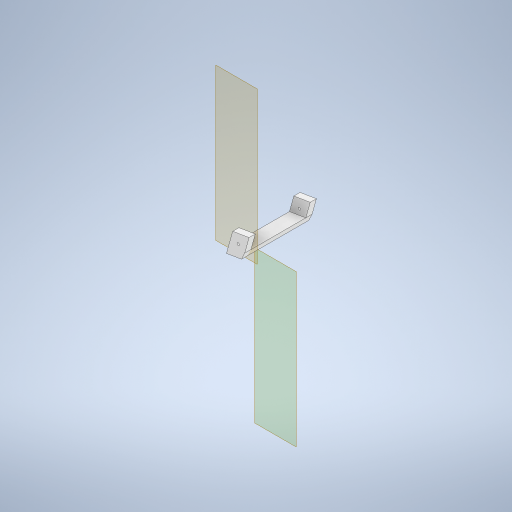
# Autodesk Inventor part: 70
Saved by Autodesk Inventor 2024.3 (Build 283343000, 343)
## iProperties
Created: 2024-09-09
Part Number: 70
Material: LCP 플라스틱
Document SubType Name: Modeling
Designer: 구지현
Density: 1.626 g/cm^3
Appearance: 흰색
Author: 구지현
Autodesk Inventor part; units mm, degrees
ref_plane "YZ Plane" through (0, 0, 0) normal (1, 0, 0) x (0, 1, 0)
ref_plane "XZ Plane" through (0, 0, 0) normal (0, 1, 0) x (-1, 0, 0)
ref_plane "XY Plane" through (0, 0, 0) normal (0, 0, 1) x (1, 0, 0)
ref_plane "작업 평면1" through (0, 0, 0) normal (0, 0, 1) x (1, 0, 0)
sketch "스케치1" plane through (0, 0, 0) normal (0, 0, 1) x (1, 0, 0)
  circle A0 centre (5.0902, -34.5274) radius 1.15 projected
  arc A1 (-17.0321, 89.7044) -> (-16.6881, 73.0594) centre (-9.9807, 81.5241) ccw projected
  line L0 (-16.6881, 73.0594) -> (-0.201, -26.5164) projected
  line L1 (-0.201, -26.5164) -> (-4.4157, -41.6132) projected
  line L2 (-4.4157, -41.6132) -> (11.3694, -38.9996) projected
  line L3 (11.3694, -38.9996) -> (15.5841, -23.9028) projected
  line L4 (15.5841, -23.9028) -> (-0.903, 75.673) projected
  arc A2 (-0.903, 75.673) -> (-5.9423, 91.5406) centre (-9.9807, 81.5241) ccw projected
  arc A3 (-5.9423, 91.5406) -> (-7.3028, 90.4498) centre (-6.3162, 90.6132) ccw projected
  line L5 (-7.3028, 90.4498) -> (-5.9358, 82.1938) projected
  arc A4 (-14.0257, 80.8544) -> (-5.9358, 82.1938) centre (-9.9807, 81.5241) ccw projected
  line L6 (-14.0257, 80.8544) -> (-15.3926, 89.1104) projected
  arc A5 (-15.3926, 89.1104) -> (-17.0321, 89.7044) centre (-16.3792, 88.947) ccw projected
  circle A6 centre (-14.6376, 75.0192) radius 1.3 projected
  circle A7 centre (-3.4758, 76.8673) radius 1.3 projected
  circle A8 centre (-5.3239, 88.029) radius 1.3 projected
  circle A9 centre (-8.6739, 73.6316) radius 1.3 projected
  circle A10 centre (-2.0882, 82.8309) radius 1.3 projected
  circle A11 centre (-16.4857, 86.1809) radius 1.3 projected
  circle A12 centre (-17.8733, 80.2173) radius 1.3 projected
  line L7 (-0.201, -26.5164) -> (15.5841, -23.9028)
  point P0 (0, 0)
  constraints: 2 end point
extrude "돌출1" add sketch "스케치1" along normal blind 6 contours L7 L3 L2 L1
ref_plane "작업 평면2" through (0, 0, -53) normal (0, 0, -1) x (-1, 0, 0)
sketch "스케치2" plane through (0, 0, -53) normal (0, 0, -1) x (-1, 0, 0)
  line L0 (4.4157, -41.6132) -> (-11.3694, -38.9996) projected
  line L1 (-11.3694, -38.9996) -> (-15.5841, -23.9028) projected
  line L2 (-15.5841, -23.9028) -> (0.201, -26.5164) projected
  line L3 (0.201, -26.5164) -> (4.4157, -41.6132) projected
  circle A0 centre (-5.0902, -34.5274) radius 1.15 projected
  point P0 (0, 0)
extrude "돌출2" add sketch "스케치2" along normal blind 6
sketch "스케치7" plane through (-4.4157, -41.6132, -59) normal (0.1633496, -0.9865682, 0) x (0.9865682, 0.1633496, 0)
  line L0 (16, 6) -> (0, 6) projected
  line L1 (0, 6) -> (0, 0) projected
  line L2 (16, 0) -> (0, 0) projected
  line L3 (16, 6) -> (16, 0) projected
  line L4 (0, 59) -> (16, 59) projected
  line L5 (16, 59) -> (16, 65) projected
  line L6 (0, 65) -> (16, 65) projected
  line L7 (0, 59) -> (0, 65) projected
  line L8 (16, 0) -> (0, 0) projected
  line L9 (0, 0) -> (16, 0)
  line L10 (16, 0) -> (16, 65)
  line L11 (16, 65) -> (0, 65)
  line L12 (0, 65) -> (0, 0)
  point P0 (11.1539, 59)
  point P1 (16, 6)
  point P2 (16, 59)
  point P3 (0, 6)
  constraints: 8 end point, 2 parallel, 1 horizontal, 1 perpendicular
extrude "돌출4" add sketch "스케치7" along normal blind 6
sketch "스케치8" plane through (0, 0, 6) normal (0, 0, 1) x (1, 0, 0)
  line L0 (11.3694, -38.9996) -> (15.5841, -23.9028) projected
  line L1 (15.5841, -23.9028) -> (-0.201, -26.5164) projected
  line L2 (-0.201, -26.5164) -> (-4.4157, -41.6132) projected
  line L3 (-4.4157, -41.6132) -> (-3.4356, -47.5326) projected
  line L4 (12.3495, -44.919) -> (-3.4356, -47.5326) projected
  line L5 (11.3694, -38.9996) -> (12.3495, -44.919) projected
  circle A0 centre (5.0902, -34.5274) radius 1.15 projected
  line L6 (11.3694, -38.9996) -> (8.2961, -45.5901)
  line L7 (11.3694, -38.9996) -> (19.8926, -38.9996) construction
  point P0 (0, 0)
  dimension "d8" = 115
  constraints: 4 end point, 1 horizontal, 1 point on line
  measures "d8" angle of L6 L7
extrude "돌출5" cut sketch "스케치8" against normal blind 70 contours L5 L4 L6
sketch "스케치9" plane through (0, 0, 6) normal (0, 0, 1) x (1, 0, 0)
  circle A0 centre (5.0902, -34.5274) radius 1.15 projected
  line L0 (8.2961, -45.5901) -> (11.3694, -38.9996) projected
  line L1 (11.3694, -38.9996) -> (15.5841, -23.9028) projected
  line L2 (15.5841, -23.9028) -> (-0.201, -26.5164) projected
  line L3 (-0.201, -26.5164) -> (-4.4157, -41.6132) projected
  line L4 (-4.4157, -41.6132) -> (-3.4356, -47.5326) projected
  line L5 (8.2961, -45.5901) -> (-3.4356, -47.5326) projected
  line L6 (-4.4157, -41.6132) -> (-7.6705, -53.2716)
  line L7 (3.9402, -46.3113) -> (-21.3119, -50.4924)
  point P0 (0, 0)
  point P1 (-6.1959, -47.9896)
  constraints: 4 end point, 2 point on line
extrude "돌출6" add sketch "스케치9" against normal blind 65 contours L7 L6 L4
